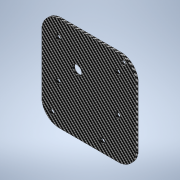
# Autodesk Inventor part: s_carbon_plate6
Saved by Autodesk Inventor 2022 (Build 260153000, 153)
## iProperties
Created: 2021-09-23
Part Number: s_carbon_plate6
Material: CFRP
Document SubType Name: Sheet Metal
Designer: yuto6
Density: 1.43 g/cm^3
Sheet Metal Rule: Default_mm
Appearance: カーボンファイバー
Author: yuto6
Autodesk Inventor part; units mm, degrees
ref_plane "YZ Plane" through (0, 0, 0) normal (1, 0, 0) x (0, 1, 0)
ref_plane "XZ Plane" through (0, 0, 0) normal (0, 1, 0) x (-1, 0, 0)
ref_plane "XY Plane" through (0, 0, 0) normal (0, 0, 1) x (1, 0, 0)
sketch "スケッチ1" plane through (0, 0, 0) normal (0, 0, 1) x (1, 0, 0)
  line L0 (40, 40) -> (-40, 40)
  line L1 (-40, 40) -> (-40, -40)
  line L2 (-40, -40) -> (40, -40)
  line L3 (40, -40) -> (40, 40)
  line L4 (40, 40) -> (-40, -40) construction
  line L5 (-40, 40) -> (40, -40) construction
  point P0 (0, 0)
  dimension "d0" = 80
  dimension "d1" = 80
  measures "d0" distance of L0.start L0.end
  measures "d1" distance of L0.end L1.end
extrude "プレート1" add sketch "スケッチ1" along normal blind 2
sketch "スケッチ8" plane through (0, 0, 2) normal (0, 0, 1) x (1, 0, 0)
  circle A0 centre (-10, 10) radius 46.5
  line L0 (24.6, 26) -> (-26, 26)
  line L1 (-26, 26) -> (-26, -6)
  line L2 (-26, -6) -> (24.6, -6)
  line L3 (24.6, -6) -> (24.6, 26)
  line L4 (24.6, 26) -> (-26, -6) construction
  line L5 (-26, 26) -> (24.6, -6) construction
  point P0 (0, 0)
  point P1 (-0.7, 10)
  point P2 (29.2078, 35)
  point P3 (11.4877, -31.2375)
  point P4 (-31.4549, -31.2545)
  dimension "d51" = 10
  dimension "d52" = 10
  dimension "d53" = 93
  dimension "d54" = 9.3
  dimension "d55" = 0
  dimension "d56" = 32
  dimension "d57" = 50.6
  dimension "d58" = 55
  dimension "d59" = 95
  dimension "d60" = 25
  constraints: 12 end point, 3 point on circle, 2 midpoint, 2 parallel, 1 centre point, 1 coincident, 1 horizontal, 1 perpendicular
  measures "d51" horizontal distance of point (0, 0) point (-10, 10)
  measures "d52" horizontal distance of point (-10, 10) point (0, 0)
  measures "d53" diameter of A0
  measures "d54" distance of A0.centre point (-0.7, 10)
  measures "d55" vertical distance of A0.centre point (-0.7, 10)
  measures "d56" distance of L0.end L1.end
  measures "d57" distance of L1.end L2.end
  measures "d60" vertical distance of A0.start A0.centre
hole "穴4" at (-26, 26, 2) at (-26, -6, 2) at (24.6, -6, 2) at (24.6, 26, 2) at (29.2078, 35, 2) at (11.4877, -31.2375, 2) at (-31.4549, -31.2545, 2) direction (0, 0, -1) diameter 4.3 end through all
hole "穴5" at (-10, 10, 2) direction (0, 0, -1) diameter 8 end through all
fillet "フィレット4" radius 15 4 edges at (40, -40, 1) (-40, -40, 1) (-40, 40, 1) (40, 40, 1)
equation "\"d2\" = Thickness"
equation "\"BendRadius\" = Thickness"
equation "\"BendReliefWidth\" = Thickness"
equation "\"BendReliefDepth\" = 0.5 * Thickness"
equation "\"CornerReliefSize\" = 4 * Thickness"
equation "\"MinimumRemnant\" = 2 * Thickness"
equation "\"TransitionRadius\" = BendRadius"
equation "\"JacobiRadiusSize\" = BendRadius"
equation "\"GapSize\" = Thickness"
equation "\"Thickness\" = 2"
